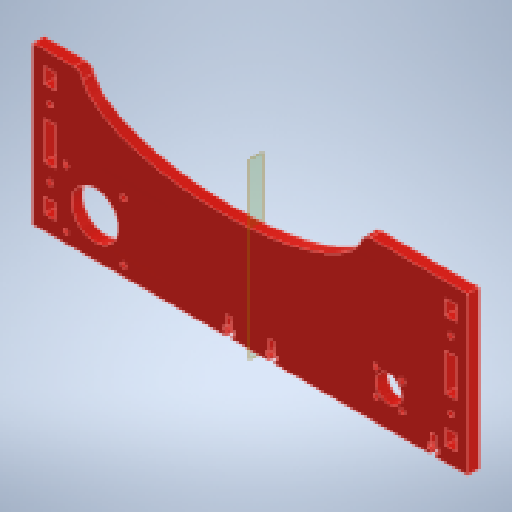
# Autodesk Inventor part: боковая стенка
Saved by Autodesk Inventor 2024.2 (Build 282272000, 272)
## iProperties
Created: 2025-11-20
Part Number: боковая стенка
Material: Типовые
Document SubType Name: Modeling
Designer: Zakhar
Density: 1 g/cm^3
Appearance: Оранжево-красный
Mass: 81.5682 g
Surface Area: 329.882 cm^2
Volume: 81.5682 cm^3
Author: Zakhar
Autodesk Inventor part; units mm, degrees
ref_plane "YZ Plane" through (0, 0, 0) normal (1, 0, 0) x (0, 1, 0)
ref_plane "XZ Plane" through (0, 0, 0) normal (0, 1, 0) x (-1, 0, 0)
ref_plane "XY Plane" through (0, 0, 0) normal (0, 0, 1) x (1, 0, 0)
sketch "Эскиз1" plane through (0, 0, 0) normal (0, 0, 1) x (1, 0, 0)
  line L0 (220, 84) -> (220, 0)
  line L1 (220, 0) -> (0, 0)
  line L2 (0, 0) -> (0, 84)
  line L3 (6, 0) -> (0, 0)
  line L4 (0, 76) -> (6, 76)
  line L5 (6, 76) -> (6, 8)
  line L6 (6, 8) -> (0, 8)
  line L7 (0, 8) -> (0, 76)
  ellipse E0 centre (95, 84) end of major axis (170, 84) minor radius 28.3094 (20, 84) -> (170, 84) ccw
  line L8 (0, 84) -> (20, 84)
  line L9 (170, 84) -> (220, 84)
  line L10 (220, 76) -> (214, 76)
  line L11 (214, 76) -> (214, 8)
  line L12 (214, 8) -> (220, 8)
  line L13 (220, 8) -> (220, 76)
  line L14 (0, 68) -> (6, 68)
  line L15 (6, 68) -> (6, 52)
  line L16 (6, 52) -> (0, 52)
  line L17 (0, 52) -> (0, 68)
  line L18 (0, 32) -> (6, 32)
  line L19 (6, 32) -> (6, 16)
  line L20 (6, 16) -> (0, 16)
  line L21 (0, 16) -> (0, 32)
  line L22 (214, 68) -> (220, 68)
  line L23 (214, 52) -> (220, 52)
  line L24 (214, 32) -> (220, 32)
  line L25 (214, 16) -> (220, 16)
  line L26 (0, 84) -> (-6, 84)
  line L27 (-6, 84) -> (-6, 0)
  line L28 (-6, 0) -> (0, 0)
  line L29 (0, 0) -> (0, 84)
  line L30 (220, 84) -> (226, 84)
  line L31 (226, 84) -> (226, 0)
  line L32 (226, 0) -> (220, 0)
  line L33 (220, 0) -> (220, 84)
  point P0 (217, 8)
  point P1 (220, 8)
  point P2 (3, 76)
  point P3 (3, 0)
  point P4 (217, 76)
  point P5 (3, 68)
  point P6 (0, 16)
  point P7 (0, 52)
  point P8 (217, 68)
  point P9 (217, 32)
  point P10 (217, 16)
  point P11 (217, 52)
  point P12 (220, 32)
  point P13 (220, 52)
  point P14 (220, 68)
  dimension "d1" = 75
  dimension "d0" = 220
  dimension "d2" = 125
  dimension "d3" = 84
  dimension "d4" = 150
  dimension "d5" = 84
  dimension "d6" = 6
  dimension "d7" = 8
  dimension "d10" = 6
  dimension "d11" = 8
  dimension "d12" = 8
  dimension "d13" = 8
  dimension "d14" = 84
  dimension "d35" = 8
  dimension "d36" = 8
  dimension "d37" = 16
  dimension "d38" = 16
  dimension "d39" = 8
  dimension "d40" = 8
  dimension "d41" = 16
  dimension "d42" = 16
  dimension "d96" = 6
  dimension "d97" = 6
  constraints: 68 end point, 15 parallel, 14 point on line, 12 perpendicular, 9 midpoint, 8 horizontal, 2 collinear, 1 coincident, 4 other
  measures "d0" distance of L1.start L1.end
  measures "d2" distance of L0.start point (95, 84)
  measures "d3" distance between parallel lines of L1 L9
  measures "d4" distance of L8.end L9.start
  measures "d5" distance from line of L1 point (95, 84)
  measures "d6" distance of L13.end L11.start
  measures "d7" vertical distance of point (217, 8) L1.start
  measures "d10" distance between parallel lines of L2 L5
  measures "d11" distance from line of L8 point (3, 76)
  measures "d12" distance from line of point (3, 0) L6
  measures "d13" distance from line of L9 point (217, 76)
  measures "d14" distance between parallel lines of L1 L8
  measures "d35" distance between parallel lines of L20 L6
  measures "d36" distance between parallel lines of L4 L14
  measures "d37" distance between parallel lines of L18 L20
  measures "d38" distance from line of point (3, 68) L16
  measures "d39" distance from line of L10 point (217, 68)
  measures "d40" distance from line of L25 point (217, 8)
  measures "d41" distance of point (217, 32) point (217, 16)
  measures "d42" distance of point (217, 68) point (217, 52)
  measures "d96" distance of L0.start L30.end
  measures "d97" distance of L8.start L26.end
extrude "Выдавливание1" add sketch "Эскиз1" along normal blind 6 contours L30 L31 L32 L0 | L0 L10 L11 L12 L1 L2 L6 L5 L4 L8 E0 L9 | L0 L23 L11 L22 | L2 L28 L27 L26 | L0 L25 L11 L24 | L14 L5 L16 L2 | L18 L5 L20 L2
sketch "Эскиз2" plane through (0, 0, 6) normal (0, 0, 1) x (1, 0, 0)
  line L0 (0, 0) -> (220, 0) projected
  line L1 (6, 0) -> (48, 0)
  line L2 (48, 0) -> (48, 8)
  line L3 (48, 8) -> (6, 8)
  line L4 (6, 8) -> (6, 0)
  line L5 (48, 0) -> (40, 0)
  line L6 (40, 0) -> (40, 42)
  line L7 (40, 42) -> (48, 42)
  line L8 (48, 42) -> (48, 0)
  line L9 (48, 42) -> (6, 42)
  line L10 (6, 42) -> (6, 34)
  line L11 (6, 34) -> (48, 34)
  line L12 (48, 34) -> (48, 42)
  line L13 (6, 42) -> (14, 42)
  line L14 (14, 42) -> (14, 0)
  line L15 (14, 0) -> (6, 0)
  line L16 (6, 0) -> (6, 42)
  line L17 (6, 16) -> (6, 8) projected
  circle A0 centre (11.5, 36.5) radius 1.5
  circle A1 centre (42.5, 36.5) radius 1.5
  circle A2 centre (42.5, 5.5) radius 1.5
  circle A3 centre (11.5, 5.5) radius 1.5
  circle A4 centre (184, 19) radius 7
  circle A5 centre (177, 25.9159) radius 1.5
  circle A6 centre (191, 26.0852) radius 1.5
  circle A7 centre (191, 12) radius 1.5
  circle A8 centre (177, 12) radius 1.5
  line L18 (177, 42.7055) -> (177, 0) construction
  line L19 (173.1146, 12) -> (210.5161, 12) construction
  line L20 (0, 0) -> (220, 0) projected
  line L21 (174.3072, 25.8833) -> (201.7049, 26.2146) construction
  line L22 (191, 29.1476) -> (191, 5.5) construction
  line L23 (214, 8) -> (214, 16) projected
  circle A9 centre (27, 21) radius 12.5
  point P0 (27, 0)
  point P1 (6, 76)
  point P2 (14, 34)
  point P3 (14, 8)
  point P4 (40, 8)
  point P5 (40, 34)
  dimension "d15" = 42
  dimension "d16" = 42
  dimension "d17" = 8
  dimension "d18" = 8
  dimension "d19" = 8
  dimension "d20" = 8
  dimension "d21" = 3
  dimension "d22" = 3
  dimension "d23" = 3
  dimension "d24" = 3
  dimension "d25" = 5.5
  dimension "d26" = 5.5
  dimension "d27" = 5.5
  dimension "d28" = 5.5
  dimension "d29" = 5.5
  dimension "d30" = 5.5
  dimension "d31" = 5.5
  dimension "d32" = 5.5
  dimension "d78" = 14
  dimension "d80" = 3
  dimension "d81" = 3
  dimension "d82" = 3
  dimension "d83" = 3
  dimension "d91" = 30
  dimension "d93" = 21
  dimension "d94" = 21
  dimension "d95" = 25
  constraints: 40 end point, 12 point on line, 10 centre point, 8 parallel, 5 horizontal, 4 perpendicular, 4 tangent, 2 vertical, 1 collinear, 1 midpoint, 1 other
  measures "d15" distance of L10.end L11.end
  measures "d16" distance of L15.end L9.end
  measures "d17" distance between parallel lines of L9 L11
  measures "d18" distance between parallel lines of L8 L6
  measures "d19" distance from line of point (27, 0) L3
  measures "d20" distance between parallel lines of L16 L14
  measures "d21" diameter of A0
  measures "d22" diameter of A1
  measures "d23" diameter of A2
  measures "d24" diameter of A3
  measures "d25" distance from line of L1 A3.centre
  measures "d26" distance from line of L16 A3.centre
  measures "d27" distance from line of L8 A2.centre
  measures "d28" distance from line of L0 A2.centre
  measures "d29" distance from line of L12 A1.centre
  measures "d30" distance from line of L7 A1.centre
  measures "d31" distance from line of L9 A0.centre
  measures "d32" distance from line of L10 A0.centre
  measures "d78" diameter of A4
  measures "d80" diameter of A5
  measures "d81" diameter of A6
  measures "d82" diameter of A7
  measures "d83" diameter of A8
  measures "d91" distance from line of L23 A4.centre
  measures "d93" distance of point (27, 0) A9.centre
  measures "d94" distance from line of L16 A9.centre
  measures "d95" diameter of A9
extrude "Выдавливание2" cut sketch "Эскиз2" against normal blind 6 contours A0 | A1 | A2 | A3 | A4 | A5 | A6 | A7 | A8 | A9
ref_plane "РабПлоскость1" through (110, 8, 0) normal (-1, 0, 0) x (0, 0, 1)
sketch "Эскиз5" plane through (0, 0, 0) normal (0, -1, 0) x (1, 0, 0)
  circle A0 centre (115, 3) radius 1.5
  circle A1 centre (105, 3) radius 1.5
  line L0 (110, -1.2) -> (110, 7.2) projected
  line L1 (0, 0) -> (220, 0) projected
  dimension "d70" = 5
  dimension "d71" = 5
  dimension "d72" = 3
  dimension "d73" = 3
  dimension "d74" = 3
  dimension "d75" = 3
  constraints: 2 centre point
  measures "d70" distance from line of L0 A1.centre
  measures "d71" distance from line of L0 A0.centre
  measures "d72" distance from line of L1 A0.centre
  measures "d73" distance from line of L1 A1.centre
  measures "d74" diameter of A1
  measures "d75" diameter of A0
extrude "Выдавливание3" [suppressed]
fillet "Сопряжение1" radius 5 2 edges at (170, 84, 3) (20, 84, 3)
sketch "Эскиз6" plane through (0, 0, 6) normal (0, 0, 1) x (1, 0, 0)
  line L0 (-6, 0) -> (226, 0) projected
  line L1 (100, 0) -> (97, 0)
  line L2 (97, 0) -> (97, 10)
  line L3 (97, 10) -> (100, 10)
  line L4 (100, 10) -> (100, 0)
  line L5 (123, 0) -> (120, 0)
  line L6 (120, 0) -> (120, 10)
  line L7 (120, 10) -> (123, 10)
  line L8 (123, 10) -> (123, 0)
  line L9 (124.5, 4.2) -> (118.5, 4.2)
  line L10 (118.5, 4.2) -> (118.5, 1.8)
  line L11 (118.5, 1.8) -> (124.5, 1.8)
  line L12 (124.5, 1.8) -> (124.5, 4.2)
  line L13 (95.5, 4.2) -> (101.5, 4.2)
  line L14 (101.5, 4.2) -> (101.5, 1.8)
  line L15 (101.5, 1.8) -> (95.5, 1.8)
  line L16 (95.5, 1.8) -> (95.5, 4.2)
  line L17 (110, -16.8) -> (110, 100.8) projected
  point P0 (0, 0)
  point P1 (120, 1.8)
  point P2 (120, 0)
  point P3 (123, 1.8)
  point P4 (123, 4.2)
  point P5 (120, 4.2)
  point P6 (97, 1.8)
  point P7 (97, 0)
  point P8 (100, 1.8)
  point P9 (100, 4.2)
  point P10 (97, 4.2)
  dimension "d98" = 10
  dimension "d99" = 10
  dimension "d100" = 13
  dimension "d101" = 3
  dimension "d102" = 3
  dimension "d103" = 10
  dimension "d104" = 6
  dimension "d105" = 8.5
  dimension "d106" = 2.4
  dimension "d107" = 1.8
  dimension "d108" = 2.4
  dimension "d109" = 6
  dimension "d110" = 8.5
  constraints: 32 end point, 8 parallel, 4 horizontal, 4 perpendicular, 3 point on line
  measures "d98" distance of L7.end L5.start
  measures "d99" distance between parallel lines of L4 L17
  measures "d100" distance between parallel lines of L8 L17
  measures "d101" distance of L6.end L7.end
  measures "d102" distance of L2.end L3.end
  measures "d103" distance between parallel lines of L0 L3
  measures "d104" distance of L14.end L15.end
  measures "d105" distance between parallel lines of L17 L14
  measures "d106" distance between parallel lines of L15 L13
  measures "d107" distance between parallel lines of L0 L15
  measures "d108" distance between parallel lines of L11 L9
  measures "d109" distance between parallel lines of L12 L10
  measures "d110" distance between parallel lines of L17 L10
extrude "Выдавливание4" cut sketch "Эскиз6" against normal blind 6
sketch "Эскиз7" plane through (0, 0, 6) normal (0, 0, 1) x (1, 0, 0)
  circle A0 centre (3, 60) radius 1.5
  circle A1 centre (3, 24) radius 1.5
  line L0 (6, 68) -> (0, 68) projected
  line L1 (6, 76) -> (6, 68) construction
  line L2 (0, 52) -> (6, 52) construction
  line L3 (6, 68) -> (6, 52) construction
  line L4 (6, 32) -> (0, 32) construction
  point P0 (0, 0)
  point P1 (3, 68)
  point P2 (3, 32)
  dimension "d113" = 3
  dimension "d114" = 3
  dimension "d115" = 8
  dimension "d116" = 3
  dimension "d118" = 8
  dimension "d119" = 3
  constraints: 2 centre point, 2 end point, 2 midpoint, 1 vertical
  measures "d113" diameter of A0
  measures "d114" diameter of A1
  measures "d115" distance of point (3, 68) A0.centre
  measures "d116" distance from line of L3 A0.centre
  measures "d118" distance from line of L4 A1.centre
  measures "d119" distance from line of L3 A1.centre
extrude "Выдавливание5" cut sketch "Эскиз7" against normal blind 6
mirror "Зеркальное отражение2" about plane through (110, 8, 0) normal (-1, 0, 0) of "Выдавливание5"
sketch "Эскиз8" plane through (0, 0, 6) normal (0, 0, 1) x (1, 0, 0)
  circle A0 centre (217, 24) radius 1.5 projected
  circle A1 centre (217, 60) radius 1.5 projected
  circle A2 centre (3, 24) radius 1.5 projected
  circle A3 centre (3, 60) radius 1.5 projected
  line L0 (0, 8) -> (0, 16) projected
  line L1 (0, 16) -> (6, 16) projected
  line L2 (6, 16) -> (6, 8) projected
  line L3 (6, 8) -> (0, 8) projected
  line L4 (0, 32) -> (0, 52) projected
  line L5 (0, 52) -> (6, 52) projected
  line L6 (6, 52) -> (6, 32) projected
  line L7 (6, 32) -> (0, 32) projected
  line L8 (0, 68) -> (0, 76) projected
  line L9 (0, 76) -> (6, 76) projected
  line L10 (6, 76) -> (6, 68) projected
  line L11 (6, 68) -> (0, 68) projected
  line L12 (220, 76) -> (220, 68) projected
  line L13 (220, 68) -> (214, 68) projected
  line L14 (214, 68) -> (214, 76) projected
  line L15 (214, 76) -> (220, 76) projected
  line L16 (220, 52) -> (220, 32) projected
  line L17 (220, 32) -> (214, 32) projected
  line L18 (214, 32) -> (214, 52) projected
  line L19 (214, 52) -> (220, 52) projected
  line L20 (220, 16) -> (220, 8) projected
  line L21 (220, 8) -> (214, 8) projected
  line L22 (214, 8) -> (214, 16) projected
  line L23 (214, 16) -> (220, 16) projected
  circle A4 centre (27, 21) radius 12.5 projected
  circle A5 centre (177, 12) radius 1.5 projected
  circle A6 centre (42.5, 5.5) radius 1.5 projected
  circle A7 centre (42.5, 36.5) radius 1.5 projected
  circle A8 centre (177, 25.9159) radius 1.5 projected
  circle A9 centre (184, 19) radius 7 projected
  circle A10 centre (191, 12) radius 1.5 projected
  circle A11 centre (11.5, 5.5) radius 1.5 projected
  circle A12 centre (11.5, 36.5) radius 1.5 projected
  circle A13 centre (191, 26.0852) radius 1.5 projected
  line L24 (120, 0) -> (120, 1.8) projected
  line L25 (120, 1.8) -> (118.5, 1.8) projected
  line L26 (118.5, 1.8) -> (118.5, 4.2) projected
  line L27 (118.5, 4.2) -> (120, 4.2) projected
  line L28 (120, 4.2) -> (120, 10) projected
  line L29 (120, 10) -> (123, 10) projected
  line L30 (123, 10) -> (123, 4.2) projected
  line L31 (123, 4.2) -> (124.5, 4.2) projected
  line L32 (124.5, 4.2) -> (124.5, 1.8) projected
  line L33 (124.5, 1.8) -> (123, 1.8) projected
  line L34 (123, 1.8) -> (123, 0) projected
  line L35 (123, 0) -> (226, 0) projected
  line L36 (226, 0) -> (226, 84) projected
  line L37 (226, 84) -> (174.1947, 84) projected
  arc A14 (174.1947, 84) -> (169.4402, 80.5476) centre (174.1947, 79) ccw projected
  ellipse E0 centre (95, 84) end of major axis (20, 84) minor radius 28.3094 (20.5598, 80.5476) -> (169.4402, 80.5476) ccw projected
  arc A15 (20.5598, 80.5476) -> (15.8053, 84) centre (15.8053, 79) ccw projected
  line L38 (15.8053, 84) -> (-6, 84) projected
  line L39 (-6, 84) -> (-6, 0) projected
  line L40 (-6, 0) -> (97, 0) projected
  line L41 (97, 0) -> (97, 1.8) projected
  line L42 (97, 1.8) -> (95.5, 1.8) projected
  line L43 (95.5, 1.8) -> (95.5, 4.2) projected
  line L44 (95.5, 4.2) -> (97, 4.2) projected
  line L45 (97, 4.2) -> (97, 10) projected
  line L46 (97, 10) -> (100, 10) projected
  line L47 (100, 10) -> (100, 4.2) projected
  line L48 (100, 4.2) -> (101.5, 4.2) projected
  line L49 (101.5, 4.2) -> (101.5, 1.8) projected
  line L50 (101.5, 1.8) -> (100, 1.8) projected
  line L51 (100, 1.8) -> (100, 0) projected
  line L52 (100, 0) -> (120, 0) projected
  line L53 (214, 58.5) -> (220, 58.5)
  line L54 (220, 58.5) -> (220, 52)
  line L55 (214, 52) -> (220, 52)
  line L56 (214, 32) -> (214, 52)
  line L57 (220, 32) -> (214, 32)
  line L58 (220, 32) -> (220, 25.5)
  line L59 (220, 25.5) -> (214, 25.5)
  line L60 (214, 25.5) -> (214, 32)
  line L61 (214, 52) -> (214, 58.5)
  line L62 (220, 52) -> (220, 32)
  line L63 (220, 61.5) -> (214, 61.5)
  line L64 (214, 61.5) -> (214, 68)
  line L65 (214, 68) -> (214, 76)
  line L66 (214, 76) -> (214, 84)
  line L67 (214, 84) -> (220, 84)
  line L68 (220, 84) -> (220, 76)
  line L69 (220, 76) -> (220, 68)
  line L70 (220, 68) -> (220, 61.5)
  line L71 (220, 68) -> (214, 68)
  line L72 (214, 76) -> (220, 76)
  line L73 (214, -6) -> (214, 8)
  line L74 (214, 8) -> (214, 16)
  line L75 (214, 16) -> (214, 22.5)
  line L76 (214, 22.5) -> (220, 22.5)
  line L77 (220, 22.5) -> (220, 16)
  line L78 (220, 16) -> (220, 8)
  line L79 (220, 8) -> (220, -6)
  line L80 (220, -6) -> (214, -6)
  line L81 (220, 8) -> (214, 8)
  line L82 (214, 16) -> (220, 16)
  line L83 (209, 0) -> (206, 0)
  line L84 (206, 0) -> (206, 10)
  line L85 (206, 10) -> (209, 10)
  line L86 (209, 10) -> (209, 0)
  line L87 (204.5, 4.4) -> (210.5, 4.4)
  line L88 (210.5, 4.4) -> (210.5, 2)
  line L89 (210.5, 2) -> (204.5, 2)
  line L90 (204.5, 2) -> (204.5, 4.4)
  point P0 (0, 0)
  point P1 (204.5, 3.2)
  point P2 (207.5, 0)
  point P3 (206, 4.4)
  point P4 (206, 2)
  point P5 (209, 2)
  point P6 (209, 4.4)
  dimension "d122" = 5
  dimension "d123" = 3
  dimension "d124" = 2.4
  dimension "d125" = 6
  dimension "d126" = 1.5
  dimension "d127" = 2
  dimension "d128" = 10
  constraints: 76 end point, 18 vertical, 14 horizontal, 4 parallel, 2 midpoint, 2 perpendicular, 1 point on line, 13 other
  measures "d122" distance between parallel lines of L73 L86
  measures "d123" distance between parallel lines of L86 L84
  measures "d124" distance between parallel lines of L89 L87
  measures "d125" distance of L88.end L89.end
  measures "d126" distance from line of L84 point (204.5, 3.2)
  measures "d127" distance between parallel lines of L35 L89
  measures "d128" distance from line of point (207.5, 0) L85
extrude "Выдавливание6" cut sketch "Эскиз8" against normal through all contours L35 L84 L89 L86 | L89 L84 L87 L86 | L86 L87 L88 L89 | L89 L90 L87 L84 | L87 L84 L85 L86
equation "\"d36\" = d35"
equation "\"d38\" = d37"
equation "\"d40\" = d39"
equation "\"d42\" = d41"
equation "\"d22\" = d21"
equation "\"d23\" = d21"
equation "\"d24\" = d21"
